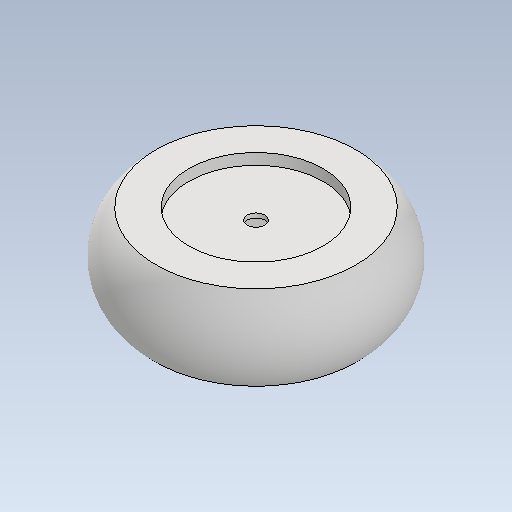
# Autodesk Inventor part: smooth-wheel
Saved by Autodesk Inventor 2025 (Build 290162000, 162)
## iProperties
Created: 2025-09-06
Part Number: smooth-wheel
Material: Generic
Document SubType Name: Modeling
Designer: HP
Density: 1 g/cm^3
Appearance: Default
Author: HP
Autodesk Inventor part; units mm, degrees
ref_plane "YZ Plane" through (0, 0, 0) normal (1, 0, 0) x (0, 1, 0)
ref_plane "XZ Plane" through (0, 0, 0) normal (0, 1, 0) x (-1, 0, 0)
ref_plane "XY Plane" through (0, 0, 0) normal (0, 0, 1) x (1, 0, 0)
sketch "Sketch1" plane through (0, 0, 0) normal (0, 0, 1) x (1, 0, 0)
  line L0 (45, 19) -> (45, -19) construction
  line L1 (45, -19) -> (30.25, -19)
  line L2 (30.25, -19) -> (30.25, 19)
  line L3 (30.25, 19) -> (45, 19)
  line L4 (45, 19) -> (30.25, -19) construction
  line L5 (45, -19) -> (30.25, 19) construction
  line L6 (4, 12) -> (4, 19)
  line L7 (4, 19) -> (30.25, 19)
  line L8 (30.25, 19) -> (30.25, 12)
  line L9 (30.25, 12) -> (4, 12)
  line L10 (4, 12) -> (30.25, 19) construction
  line L11 (4, 19) -> (30.25, 12) construction
  arc A0 (45, -19) -> (45, 19) centre (28.7519, 0) ccw
  line L12 (30.25, 14) -> (4, 14)
  line L13 (0, -26.6) -> (0, 26.6) projected
  point P0 (0, 0)
  point P1 (37.625, 0)
  point P2 (17.125, 15.5)
  dimension "d0" = 45
  dimension "d1" = 38
  dimension "d2" = 4
  dimension "d3" = 30.25
  dimension "d4" = 5
  dimension "d5" = 2
  dimension "d6" = 25
  constraints: 26 end point, 4 midpoint, 4 parallel, 3 perpendicular, 2 collinear, 2 point on circle, 2 point on line, 1 centre point, 1 horizontal, 1 horizontal alignment
  measures "d0" distance from line of point (0, 0) L0
  measures "d1" distance between parallel lines of L1 L3
  measures "d2" distance from line of point (0, 0) L6
  measures "d3" distance from line of point (0, 0) L2
  measures "d4" distance between parallel lines of L12 L7
  measures "d5" distance between parallel lines of L12 L9
  measures "d6" radius of A0
revolve "Revolution1" add sketch "Sketch1" angle 360 about axis through (0, -10, 0) along (0, 1, 0) contours L1 L2 L3 A0 | L9 L6 L12 L2
body "Solid1"
